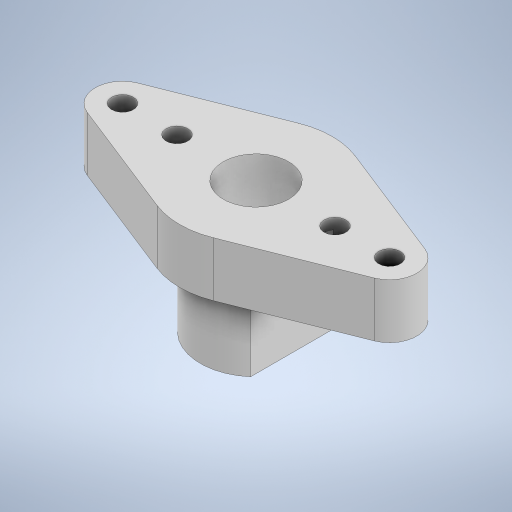
# Autodesk Inventor part: stick
Saved by Autodesk Inventor 2023 (Build 270158000, 158)
## iProperties
Created: 2023-01-25
Part Number: stick
Material: 一般
Document SubType Name: Modeling
Designer: taka2
Density: 1 g/cm^3
Appearance: 既定
Author: taka2
Autodesk Inventor part; units mm, degrees
ref_plane "YZ Plane" through (0, 0, 0) normal (1, 0, 0) x (0, 1, 0)
ref_plane "XZ Plane" through (0, 0, 0) normal (0, 1, 0) x (-1, 0, 0)
ref_plane "XY Plane" through (0, 0, 0) normal (0, 0, 1) x (1, 0, 0)
sketch "スケッチ1" plane through (0, 0, 0) normal (0, 1, 0) x (-1, 0, 0)
  arc A0 (-1.75, -3.0311) -> (-1.75, 3.0311) centre (0, 0) ccw
  arc A1 (-3.35, -3.8455) -> (-3.35, 3.8455) centre (0, 0) ccw
  line L0 (-1.75, 3.0311) -> (-1.75, -3.0311)
  line L1 (-3.35, 3.8455) -> (-3.35, -3.8455)
  point P0 (-1.75, 0)
  point P1 (3.5, 0)
  dimension "d0" = 7
  dimension "d1" = 1.6
  dimension "d3" = 1.6
  dimension "d21" = 5.25
  constraints: 5 point on circle, 4 end point, 2 centre point, 2 coincident, 2 vertical, 1 midpoint
  measures "d0" diameter of A0
  measures "d1" radial gap between concentric circles of A1 A0
  measures "d3" distance between parallel lines of L1 L0
  measures "d21" distance of point (-1.75, 0) point (3.5, 0)
extrude "押し出し1" add sketch "スケッチ1" against normal blind 7
sketch "スケッチ2" plane through (0, 0, 0) normal (0, 1, 0) x (-1, 0, 0)
  circle A0 centre (0, 0) radius 3
  circle A1 centre (7.25, 0) radius 1
  circle A2 centre (12.25, 0) radius 1
  line L0 (21.35, 0) -> (-16.3472, 0)
  line L1 (-21.4194, 0) -> (25.6478, 0)
  line L2 (0, 13.6596) -> (0, -18.5916)
  circle A3 centre (-7.25, 0) radius 1
  circle A4 centre (-12.25, 0) radius 1
  arc A5 (13.1684, -2.3252) -> (13.1684, 2.3252) centre (12.25, 0) ccw
  line L3 (13.1684, 2.3252) -> (2.5714, 6.5106)
  line L4 (13.1684, -2.3252) -> (2.5714, -6.5106)
  arc A6 (-13.1684, 2.3252) -> (-13.1684, -2.3252) centre (-12.25, 0) ccw
  line L5 (-13.1684, 2.3252) -> (-2.5714, 6.5106)
  line L6 (-13.1684, -2.3252) -> (-2.5714, -6.5106)
  arc A7 (-2.5714, -6.5106) -> (2.5714, -6.5106) centre (0, 0) ccw
  arc A8 (2.5714, 6.5106) -> (-2.5714, 6.5106) centre (0, 0) ccw
  circle A9 centre (0, 0) radius 5.5
  circle A10 centre (0, 0) radius 6.5
  dimension "d6" = 6
  dimension "d7" = 7.25
  dimension "d8" = 5
  dimension "d9" = 2
  dimension "d11" = 5
  dimension "d12" = 7
  dimension "d17" = 11
  dimension "d18" = 13
  constraints: 14 end point, 11 centre point, 9 symmetric about line, 8 point on circle, 6 point on line, 5 coincident, 2 horizontal, 2 tangent, 1 equal radius, 1 vertical, 3 other
  measures "d6" diameter of A0
  measures "d7" distance of A1.centre point (0, 0)
  measures "d8" distance of A1.centre A2.centre
  measures "d9" diameter of A1
  measures "d11" diameter of A5
  measures "d12" radius of A7
  measures "d17" diameter of A9
  measures "d18" diameter of A10
extrude "押し出し2" add sketch "スケッチ2" along normal blind 1 contours L0 A9 L2 A0 | A0 L2 A9 L0 | A0 L0 A9 L2 | L2 A9 L0 A0 | A9 L2 A10 A1 L0 | L0 A1 A10 L2 A9 | A9 L0 A3 A10 L2 | L2 A10 A3 L0 A9 | L0 A10 A1 | A1 A10 L0 | A10 A3 L0 A4 A6 L5 A8 L2 | L2 A8 L3 A5 L0 A2 A1 A10 | A10 A1 L0 A2 A5 L4 A7 L2 | L2 A7 L6 A6 L0 A4 A3 A10 | A1 L0 A10 | A10 L0 A1 | A3 A10 L0 | L0 A10 A3 | A10 L0 A3 | A3 L0 A10 | L0 A2 | A2 L0 | A4 L0 | L0 A4
extrude "押し出し3" add sketch "スケッチ2" along normal blind 5 contours L0 A9 L2 A0 | A0 L2 A9 L0 | A0 L0 A9 L2 | L2 A9 L0 A0 | A9 L2 A10 A1 L0 | L0 A1 A10 L2 A9 | A9 L0 A3 A10 L2 | L2 A10 A3 L0 A9 | A10 A3 L0 A4 A6 L5 A8 L2 | L2 A8 L3 A5 L0 A2 A1 A10 | A10 A1 L0 A2 A5 L4 A7 L2 | L2 A7 L6 A6 L0 A4 A3 A10
extrude "押し出し4" cut sketch "スケッチ2" along normal blind 4 contours A9 L2 A10 A1 L0 | L0 A1 A10 L2 A9 | A9 L0 A3 A10 L2 | L2 A10 A3 L0 A9 | L0 A10 A1 | A1 A10 L0 | A3 A10 L0 | L0 A10 A3 picked at (6.3418, -0.0745) picked at (6.3418, 0.0745) picked at (-6.3418, -0.0745) picked at (-6.3418, 0.0745)
